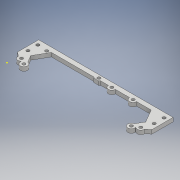
# Autodesk Inventor part: 2-4枚目
Saved by Autodesk Inventor 2018 (Build 220112000, 112)
## iProperties
Created: 2018-08-16
Part Number: 2-4枚目
Material: 一般
Document SubType Name: Modeling
Designer: shun2
Density: 1 g/cm^3
Appearance: 既定
Author: shun2
Autodesk Inventor part; units mm, degrees
ref_plane "YZ Plane" through (0, 0, 0) normal (1, 0, 0) x (0, 1, 0)
ref_plane "XZ Plane" through (0, 0, 0) normal (0, 1, 0) x (-1, 0, 0)
ref_plane "XY Plane" through (0, 0, 0) normal (0, 0, 1) x (1, 0, 0)
sketch "スケッチ1" plane through (0, 0, 0) normal (0, 0, 1) x (1, 0, 0)
  line L0 (176.2009, 5.8345) -> (176.6082, 6.0336)
  arc A0 (176.6082, 6.0336) -> (184.6641, 10.5188) centre (179.6946, 9.9674) ccw
  line L1 (190.3548, 14.9674) -> (184.6641, 10.5188)
  line L2 (35.1774, 38.4674) -> (24.4964, 38.4674)
  line L3 (24.4964, 38.4674) -> (13.8155, 19.9674)
  line L4 (13.8155, 19.9674) -> (19.605, 9.9396)
  line L5 (165.8584, 38.4674) -> (176.5394, 19.9674)
  line L6 (176.5394, 19.9674) -> (170.7498, 9.9396)
  circle A1 centre (179.6946, 9.9674) radius 2.15
  line L7 (190.3548, 44.9674) -> (190.3548, 14.9674)
  line L8 (14.154, 5.8345) -> (13.7466, 6.0336)
  arc A2 (5.6908, 10.5188) -> (13.7466, 6.0336) centre (10.6603, 9.9674) ccw
  line L9 (0, 14.9674) -> (5.6908, 10.5188)
  circle A3 centre (10.6603, 9.9674) radius 2.15
  line L10 (0, 44.9674) -> (0, 14.9674)
  line L11 (35.1774, 38.4674) -> (85.1633, 38.4674)
  line L12 (94.1916, 38.4674) -> (105.1774, 38.4674)
  line L13 (115.1774, 38.4674) -> (135.1774, 38.4674)
  line L14 (145.1774, 38.4674) -> (165.8584, 38.4674)
  line L15 (0, 44.9674) -> (190.3548, 44.9674)
  circle A4 centre (89.6774, 40.6174) radius 2.15
  arc A5 (93.2481, 37.1174) -> (94.1916, 38.4674) centre (89.6774, 40.6174) ccw
  arc A6 (85.1633, 38.4674) -> (86.1067, 37.1174) centre (89.6774, 40.6174) ccw
  circle A7 centre (110.1774, 38.4674) radius 2.15
  arc A8 (105.1774, 38.4674) -> (115.1774, 38.4674) centre (110.1774, 38.4674) ccw
  circle A9 centre (140.1774, 38.4674) radius 2.15
  arc A10 (135.1774, 38.4674) -> (145.1774, 38.4674) centre (140.1774, 38.4674) ccw
  circle A11 centre (171.2766, 4.9674) radius 2.15
  arc A12 (170.7498, 9.9396) -> (176.2009, 5.8345) centre (171.2766, 4.9674) ccw
  circle A13 centre (19.0782, 4.9674) radius 2.15
  arc A14 (14.154, 5.8345) -> (19.605, 9.9396) centre (19.0782, 4.9674) ccw
  line L16 (86.1067, 37.1174) -> (93.2481, 37.1174)
  circle A15 centre (19.2933, 36.9735) radius 2.15
  circle A16 centre (5.8155, 23.9674) radius 2.15
  circle A17 centre (5.8155, 37.9674) radius 2.15
  circle A18 centre (184.5394, 23.9674) radius 2.15
  circle A19 centre (184.5394, 37.9674) radius 2.15
  line L17 (0, 44.9674) -> (190.3548, 44.9674)
  line L18 (190.3548, 44.9674) -> (190.3548, 14.9674)
  line L19 (0, 14.9674) -> (0, 44.9674)
  line L20 (184.6641, 10.5188) -> (190.3548, 14.9674)
  line L21 (0, 14.9674) -> (5.6908, 10.5188)
  line L22 (13.8155, 19.9674) -> (24.4964, 38.4674)
  line L23 (85.1633, 38.4674) -> (24.4964, 38.4674)
  line L24 (115.1774, 38.4674) -> (135.1774, 38.4674)
  line L25 (145.1774, 38.4674) -> (165.8584, 38.4674)
  line L26 (170.7498, 9.9396) -> (176.5394, 19.9674)
  line L27 (19.605, 9.9396) -> (13.8155, 19.9674)
  line L28 (13.7466, 6.0336) -> (14.154, 5.8345)
  line L29 (176.6082, 6.0336) -> (176.2009, 5.8345)
  arc A20 (5.6908, 10.5188) -> (13.7466, 6.0336) centre (10.6603, 9.9674) ccw
  arc A21 (14.154, 5.8345) -> (19.605, 9.9396) centre (19.0782, 4.9674) ccw
  arc A22 (170.7498, 9.9396) -> (176.2009, 5.8345) centre (171.2766, 4.9674) ccw
  arc A23 (176.6082, 6.0336) -> (184.6641, 10.5188) centre (179.6946, 9.9674) ccw
  arc A24 (135.1774, 38.4674) -> (145.1774, 38.4674) centre (140.1774, 38.4674) ccw
  arc A25 (105.1774, 38.4674) -> (115.1774, 38.4674) centre (110.1774, 38.4674) ccw
  arc A26 (93.2481, 37.1174) -> (94.1916, 38.4674) centre (89.6774, 40.6174) ccw
  arc A27 (85.1633, 38.4674) -> (86.1067, 37.1174) centre (89.6774, 40.6174) ccw
  line L30 (86.1067, 37.1174) -> (93.2481, 37.1174)
  circle A28 centre (5.8155, 37.9674) radius 2.15
  circle A29 centre (19.2933, 36.9735) radius 2.15
  circle A30 centre (5.8155, 23.9674) radius 2.15
  circle A31 centre (10.6603, 9.9674) radius 2.15
  circle A32 centre (19.0782, 4.9674) radius 2.15
  circle A33 centre (89.6774, 40.6174) radius 2.15
  circle A34 centre (110.1774, 38.4674) radius 2.15
  circle A35 centre (140.1774, 38.4674) radius 2.15
  circle A36 centre (184.5394, 37.9674) radius 2.15
  circle A37 centre (184.5394, 23.9674) radius 2.15
  circle A38 centre (179.6946, 9.9674) radius 2.15
  circle A39 centre (171.2766, 4.9674) radius 2.15
  line L31 (0, 44.9674) -> (190.3548, 44.9674)
  line L32 (190.3548, 44.9674) -> (190.3548, 14.9674)
  line L33 (190.3548, 14.9674) -> (184.6641, 10.5188)
  line L34 (0, 44.9674) -> (0, 14.9674)
  line L35 (5.6908, 10.5188) -> (0, 14.9674)
  line L36 (24.4964, 38.4674) -> (13.8155, 19.9674)
  line L37 (19.605, 9.9396) -> (13.8155, 19.9674)
  line L38 (24.4964, 38.4674) -> (85.1633, 38.4674)
  line L39 (94.1916, 38.4674) -> (105.1774, 38.4674)
  line L40 (115.1774, 38.4674) -> (135.1774, 38.4674)
  line L41 (145.1774, 38.4674) -> (165.8584, 38.4674)
  line L42 (165.8584, 38.4674) -> (176.5394, 19.9674)
  line L43 (176.5394, 19.9674) -> (170.7498, 9.9396)
  point P0 (0, 0)
  constraints: 88 end point, 40 centre point, 33 point on circle, 18 concentric, 17 collinear, 12 coincident, 6 point on line, 3 perpendicular, 2 parallel, 1 horizontal
sketch "スケッチ2" plane through (0, 0, 0) normal (0, 0, 1) x (1, 0, 0)
  point P0 (0, 0)
extrude "押し出し1" add sketch "スケッチ1" along normal blind 5.5
